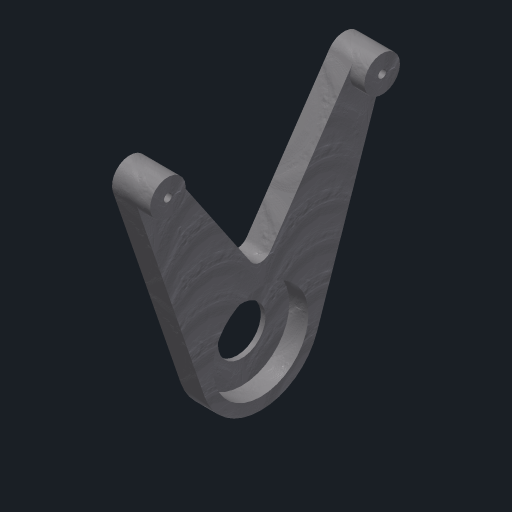
# Autodesk Inventor part: SOPORTE_RODAMIENTO
Saved by Autodesk Inventor 2024.3 (Build 283343000, 343)
## iProperties
Created: 2024-07-12
Part Number: SOPORTE_RODAMIENTO
Material: Steel, Mild, Welded
Document SubType Name: Modeling
Designer: Niler
Density: 7.85 g/cm^3
Appearance: Weld - Steel Mild
Author: Niler
Autodesk Inventor part; units mm, degrees
ref_plane "YZ Plane" through (0, 0, 0) normal (1, 0, 0) x (0, 1, 0)
ref_plane "XZ Plane" through (0, 0, 0) normal (0, 1, 0) x (-1, 0, 0)
ref_plane "XY Plane" through (0, 0, 0) normal (0, 0, 1) x (1, 0, 0)
sketch "Sketch1" plane through (0, 0, 0) normal (1, 0, 0) x (0, 1, 0)
  circle A0 centre (0, 0) radius 90 construction
  circle A1 centre (0, 0) radius 10
  circle A2 centre (0, 0) radius 25
  line L0 (77.9423, 45) -> (77.9423, -45) construction
  line L1 (-8.0516, 23.668) -> (75.5268, 52.1004)
  circle A3 centre (77.9423, 45) radius 1.65
  circle A4 centre (77.9423, 45) radius 7.5
  line L2 (82.1544, 38.7945) -> (25, 0)
  line L3 (0, 0) -> (51.9077, 0)
  line L4 (-8.0516, -23.668) -> (75.5268, -52.1004)
  circle A5 centre (77.9423, -45) radius 1.65
  circle A6 centre (77.9423, -45) radius 7.5
  line L5 (82.1544, -38.7945) -> (25, 0)
  point P0 (77.9423, 0)
  dimension "d0" = 180
  dimension "d1" = 20
  dimension "d2" = 50
  dimension "d3" = 90
  dimension "d4" = 3.3
  dimension "d5" = 15
  constraints: 12 end point, 8 point on circle, 7 centre point, 7 coincident, 5 symmetric about line, 3 tangent, 1 horizontal, 1 horizontal alignment, 1 midpoint, 2 other
  measures "d0" diameter of A0
  measures "d1" diameter of A1
  measures "d2" diameter of A2
  measures "d3" distance of L0.start L0.end
  measures "d4" diameter of A3
  measures "d5" diameter of A4
extrude "Extrusion1" add sketch "Sketch1" along normal blind 10
fillet "Fillet1" radius 5 1 edges at (5, 25, 0)
sketch "Sketch2" plane through (10, 0, 0) normal (1, 0, 0) x (0, 0, -1)
  circle A0 centre (0, 0) radius 10 projected
  circle A1 centre (0, 0) radius 20
  dimension "d9" = 40
  constraints: 1 centre point, 1 coincident
  measures "d9" diameter of A1
extrude "Extrusion2" cut sketch "Sketch2" against normal blind 8
sketch "Sketch3" plane through (10, 0, 0) normal (1, 0, 0) x (0, 0, -1)
  circle A0 centre (0, 0) radius 20 projected
  arc A1 (-38.7945, 82.1544) -> (-52.1004, 75.5268) centre (-45, 77.9423) ccw projected
  line L0 (-52.1004, 75.5268) -> (-23.668, -8.0516) projected
  arc A2 (-23.668, -8.0516) -> (23.668, -8.0516) centre (0, 0) ccw projected
  line L1 (23.668, -8.0516) -> (52.1004, 75.5268) projected
  arc A3 (52.1004, 75.5268) -> (38.7945, 82.1544) centre (45, 77.9423) ccw projected
  line L2 (38.7945, 82.1544) -> (4.137, 31.0949) projected
  arc A4 (-4.137, 31.0949) -> (4.137, 31.0949) centre (0, 33.9029) ccw projected
  line L3 (-4.137, 31.0949) -> (-38.7945, 82.1544) projected
  circle A5 centre (45, 77.9423) radius 1.65 projected
  circle A6 centre (-45, 77.9423) radius 1.65 projected
  circle A7 centre (-45, 77.9423) radius 7.5
  circle A8 centre (45, 77.9423) radius 7.5
  point P0 (38.7945, 82.1544)
  point P1 (52.1004, 75.5268)
  point P2 (-52.1004, 75.5268)
  constraints: 2 centre point, 2 coincident, 2 concentric
extrude "Extrusion3" add sketch "Sketch3" along normal blind 6 contours A7 A1 | A3 A8
body "Solid1"
